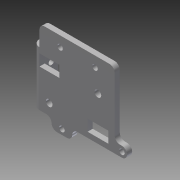
# Autodesk Inventor part: hook mount plate
Saved by Autodesk Inventor 2013 (Build 170138000, 138)
## iProperties
Created: 2013-01-27
Part Number: hook mount plate
Material: Steel
Document SubType Name: Sheet Metal
Designer: Arpan
Density: 7.85 g/cm^3
Sheet Metal Rule: Default
Mass: 318.43 g
Surface Area: 168.381 cm^2
Volume: 40.5643 cm^3
Author: Arpan
Autodesk Inventor part; units mm, degrees
ref_plane "YZ Plane" through (0, 0, 0) normal (1, 0, 0) x (0, 1, 0)
ref_plane "XZ Plane" through (0, 0, 0) normal (0, 1, 0) x (-1, 0, 0)
ref_plane "XY Plane" through (0, 0, 0) normal (0, 0, 1) x (1, 0, 0)
sketch "Sketch1" plane through (0, 0, 0) normal (0, 0, 1) x (1, 0, 0)
  line L0 (80.7, -46.515) -> (80.7, -60.485)
  line L1 (80.7, -60.485) -> (55.3, -60.485)
  line L2 (55.3, -60.485) -> (55.3, -46.515)
  line L3 (55.3, -46.515) -> (80.7, -46.515)
  line L4 (-4.699, -6.5024) -> (20.701, -6.5024)
  line L5 (20.701, -6.5024) -> (20.701, -20.4724)
  line L6 (20.701, -20.4724) -> (-4.699, -20.4724)
  line L7 (-4.699, -20.4724) -> (-4.699, -6.5024)
  circle A0 centre (8, -53.5) radius 4.15
  circle A1 centre (68, -13.5) radius 4.15
  line L8 (25.3, 0) -> (-12.7, 0)
  line L9 (-12.7, 0) -> (-12.7, -67)
  line L10 (-12.7, -67) -> (41.175, -67)
  line L11 (66.575, -67) -> (88.7, -67)
  line L12 (88.7, 0) -> (50.7, 0)
  line L13 (66.575, -67) -> (41.175, -67)
  line L14 (25.3, 0) -> (50.7, 0)
  line L15 (38, -67) -> (23.7125, -67)
  line L16 (23.7125, -67) -> (36.4125, -67)
  line L17 (36.4125, -67) -> (36.4125, -79.7)
  line L18 (36.4125, -79.7) -> (11.0125, -79.7)
  line L19 (11.0125, -79.7) -> (11.0125, -67)
  line L20 (23.7125, -67) -> (23.7125, -73.35)
  circle A2 centre (23.7125, -73.35) radius 3.3782
  line L21 (88.7, 0) -> (82.35, 0)
  line L22 (88.7, -67) -> (103.94, -67)
  line L23 (103.94, -67) -> (103.94, -54.3)
  line L24 (103.94, -54.3) -> (88.7, -54.3)
  line L25 (88.7, -54.3) -> (88.7, -67)
  line L26 (88.7, -60.65) -> (97.59, -60.65)
  circle A3 centre (97.59, -60.65) radius 3.3782
  line L27 (88.7, 0) -> (88.7, -54.3)
  point P0 (0, 0)
  point P1 (76, 0)
  dimension "d0" = 14.2875
  dimension "d1" = 12.7
  dimension "d2" = 12.7
  dimension "d3" = 25.4
  dimension "d4" = 6.35
  dimension "d5" = 6.7564
  dimension "d11" = 6.35
  dimension "d23" = 15.24
  dimension "d24" = 12.7
  dimension "d25" = 8.89
  dimension "d26" = 6.7564
  measures "d0" distance of L15.start L15.end
  measures "d1" distance of L15.end L16.end
  measures "d2" distance of L16.end L17.end
  measures "d3" distance of L17.end L18.end
  measures "d4" distance of L15.end L20.end
  measures "d5" diameter of A2
  measures "d11" distance of L12.start L21.end
  measures "d23" distance of L11.end L22.end
  measures "d24" distance of L22.end L23.end
  measures "d25" distance of L26.start L26.end
  measures "d26" diameter of A3
extrude "Plate1" add sketch "Sketch1" along normal blind 6.35
sketch "Sketch2" plane through (-6.35, 0, 6.35) normal (-1, 0, 0) x (0, -1, 0)
  line L0 (67, 0) -> (0, 0)
  line L1 (0, 0) -> (0, -25.4)
  line L2 (0, -25.4) -> (67, -25.4)
  line L3 (67, -25.4) -> (67, 0)
  constraints: 6 end point, 1 horizontal, 1 perpendicular, 1 vertical
edge flange "Flange1" height 25.4 angle 90 thickness 6.35 bend radius 2.45 thickness toward (-1, 0, 0) relief straight relief width 6.35 relief depth 3.175 edges at (-12.7, -33.5, 0) wall of the first edge with corners at (-6.35, -67, 6.35) (-6.35, 0, 6.35) (-6.35, 0, -19.05) (-6.35, -67, -19.05)
bend "Bend1"
corner "Corner1"
sketch "Sketch3" plane through (-12.7, -67, -19.05) normal (-1, 0, 0) x (0, 0, 1)
  line L0 (0, 67) -> (16.6, 67) projected
  line L1 (16.6, 0) -> (0, 0) projected
  line L2 (8.3, 67) -> (8.3, 41.6)
  line L3 (8.3, 41.6) -> (8.3, 16.2)
  circle A0 centre (8.3, 41.6) radius 3.3782
  circle A1 centre (8.3, 16.2) radius 3.3782
  point P0 (19.05, 67)
  dimension "d37" = 25.4
  dimension "d38" = 25.4
  dimension "d39" = 6.7564
  dimension "d40" = 6.7564
  constraints: 4 end point, 2 centre point, 2 coincident, 1 collinear, 1 midpoint, 1 perpendicular
  measures "d37" distance of L2.start L2.end
  measures "d38" distance of L2.end L3.end
  measures "d39" diameter of A0
  measures "d40" diameter of A1
extrude "Cut1" cut sketch "Sketch3" against normal blind 6.35
sketch "Sketch4" plane through (0, 0, 0) normal (0, 0, -1) x (-1, 0, 0)
  line L0 (-88.7, 0) -> (3.9, 0)
  line L1 (3.9, 0) -> (3.9, 25.4)
  line L2 (3.9, 25.4) -> (-89.88, 25.4)
  line L3 (-89.88, 25.4) -> (-89.88, 0)
  line L4 (-89.88, 12.7) -> (-64.48, 12.7)
  line L5 (3.9, 12.7) -> (-21.5, 12.7)
  circle A0 centre (-21.5, 12.7) radius 3.3782
  line L6 (-89.88, 0) -> (3.9, 0)
  circle A1 centre (-64.48, 12.7) radius 3.3782
  point P0 (0, 0)
  dimension "d43" = 25.4
  dimension "d44" = 25.4
  dimension "d45" = 25.4
  dimension "d47" = 6.7564
  dimension "d48" = 0
  dimension "d54" = 6.7564
  measures "d43" distance of L1.start L1.end
  measures "d44" distance of L4.start L4.end
  measures "d45" distance of L5.start L5.end
  measures "d47" diameter of A0
  measures "d48" distance from line of L0.end L1
  measures "d54" diameter of A1
sheet face with bend "Face2" sketch "Sketch4" thickness 6.35 toward (0, 0, 1) bend radius 6.35 relief straight relief width 6.35 relief depth 3.175
bend "Bend2"
sketch "Sketch5" plane through (0, 0, 6.35) normal (0, 0, 1) x (1, 0, 0)
  line L0 (89.88, 0) -> (88.7, 0) projected
  line L1 (89.88, 25.4) -> (89.88, 0) projected
  line L2 (-3.9, 25.4) -> (89.88, 25.4) projected
  line L3 (88.7, 0) -> (88.7, 25.4)
  point P0 (0, 0)
  constraints: 2 end point, 1 perpendicular, 1 point on line
extrude "Cut2" cut sketch "Sketch5" against normal blind 6.35
fillet "Corner Round1" radius 6.35 11 edges at (-3.9, 25.4, 3.175) (88.7, 25.4, 3.175) (88.7, -54.3, 3.175) (103.94, -54.3, 3.175) (103.94, -67, 3.175) (11.0125, -79.7, 3.175) (36.4125, -79.7, 3.175) (36.4125, -67, 3.175) (11.0125, -67, 3.175) (-9.525, -67, -19.05) (-9.525, 0, -19.05)
equation "\"d41\" = Thickness"
equation "\"d55\" = Thickness"
equation "\"d27\" = BendReliefWidth"
equation "\"d28\" = BendReliefDepth"
equation "\"d29\" = MinimumRemnant"
equation "\"d30\" = BendRadius"
equation "\"d34\" = CornerReliefSize"
equation "\"d35\" = GapSize"
equation "\"d36\" = JacobiRadiusSize"
equation "\"d49\" = BendRadius"
equation "\"d50\" = BendReliefWidth"
equation "\"d52\" = MinimumRemnant"
equation "\"d51\" = BendReliefDepth"
equation "\"d53\" = BendRadius"
equation "\"BendRadius\" = Thickness"
equation "\"BendReliefWidth\" = Thickness"
equation "\"BendReliefDepth\" = 0.5 * Thickness"
equation "\"CornerReliefSize\" = 4 * Thickness"
equation "\"MinimumRemnant\" = 2 * Thickness"
equation "\"TransitionRadius\" = BendRadius"
equation "\"JacobiRadiusSize\" = BendRadius"
equation "\"GapSize\" = Thickness"
equation "\"d16\" = BendRadius"
equation "\"Thickness\" = 6.35"
body "Solid1"
